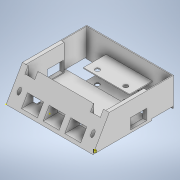
# Autodesk Inventor part: Base Onixium2
Saved by Autodesk Inventor 2021 (Build 250183000, 183)
## iProperties
Created: 2021-10-26
Part Number: Base Onixium2
Material: Genérico
Document SubType Name: Chapa
Designer: Juan Camilo
Density: 1 g/cm^3
Sheet Metal Rule: Por defecto_mm
Appearance: Valor por defecto
Author: Juan Camilo
Autodesk Inventor part; units mm, degrees
ref_plane "YZ Plane" through (0, 0, 0) normal (1, 0, 0) x (0, 1, 0)
ref_plane "XZ Plane" through (0, 0, 0) normal (0, 1, 0) x (-1, 0, 0)
ref_plane "XY Plane" through (0, 0, 0) normal (0, 0, 1) x (1, 0, 0)
sketch "Boceto2" plane through (0, 0, 0) normal (0, 1, 0) x (-1, 0, 0)
  line L0 (-49, 0) -> (49, 0)
  line L1 (49, 0) -> (49, -87)
  line L2 (49, -87) -> (-49, -87)
  line L3 (-49, -87) -> (-49, 0)
  line L4 (0, -87) -> (0, 0) construction
  circle A0 centre (-41.5, -7.5) radius 1.75
  circle A1 centre (41.5, -7.5) radius 1.75
  line L5 (-26, -87) -> (-26, -66)
  line L6 (-26, -66) -> (-49, -66)
  line L7 (26, -87) -> (26, -66)
  line L8 (26, -66) -> (49, -66)
  line L9 (49, -12) -> (-49, -12) construction
  line L10 (44.5, -24.05) -> (28.5, -24.05)
  line L11 (28.5, -24.05) -> (28.5, -13.05)
  line L12 (28.5, -13.05) -> (44.5, -13.05)
  line L13 (44.5, -13.05) -> (44.5, -24.05)
  line L14 (42.5, -23.55) -> (31.5, -23.55)
  line L15 (31.5, -14.85) -> (42.5, -14.85)
  line L16 (42.5, -14.85) -> (42.5, -23.55)
  circle A2 centre (30.2, -19.25) radius 1.05
  line L17 (31.5, -14.85) -> (31.5, -23.55)
  line L18 (-42.5, -23.55) -> (-31.5, -23.55)
  line L19 (-31.5, -14.85) -> (-42.5, -14.85)
  line L20 (-42.5, -14.85) -> (-42.5, -23.55)
  circle A3 centre (-30.2, -19.25) radius 1.05
  line L21 (-31.5, -14.85) -> (-31.5, -23.55)
  circle A4 centre (13, -21.5) radius 2.5
  circle A5 centre (-13, -21.5) radius 2.5
  circle A6 centre (16, -70) radius 2.5
  circle A7 centre (-16, -70) radius 2.5
  point P0 (26, -87)
  dimension "d6" = 3.5
  dimension "d210" = 0
  dimension "d219" = 87
  dimension "d220" = 21
  dimension "d221" = 12
  dimension "d222" = 23
  dimension "d223" = 98
  dimension "d224" = 7.5
  dimension "d225" = 7.5
  dimension "d226" = 79.5
  dimension "d229" = 2.1
  dimension "d230" = 9
  dimension "d231" = 11
  dimension "d232" = 16
  dimension "d235" = 1
  dimension "d236" = 3.6
  dimension "d239" = 2.1
  dimension "d241" = 1.3
  dimension "d242" = 5
  dimension "d243" = 36
  dimension "d244" = 9.5
  dimension "d245" = 5
  dimension "d246" = 17
  dimension "d247" = 10
  dimension "d252" = 8.7
  dimension "d254" = 4.3
  dimension "d255" = 4
  dimension "d256" = 11
  dimension "d257" = 54
  dimension "d258" = 2.85
  constraints: 44 end point, 10 symmetric about line, 8 centre point, 5 parallel, 5 point on line, 4 horizontal, 4 perpendicular, 3 midpoint, 1 equal radius, 1 vertical, 3 other
  measures "d6" diameter of A0
  measures "d210" distance of point (0, 0) L4.end
  measures "d219" distance of L1.start L1.end
  measures "d220" distance of L7.start L8.start
  measures "d221" distance between parallel lines of L0 L9
  measures "d222" distance of L8.start L8.end
  measures "d223" distance of L0.start L1.start
  measures "d224" distance from line of L1 A1.centre
  measures "d225" distance from line of L0 A1.centre
  measures "d229" diameter of L9 L12
  measures "d230" diameter of L1 L13
  measures "d231" distance of L10.end L11.end
  measures "d232" distance of L10.start L10.end
  measures "d235" diameter of L14 L10
  measures "d236" diameter of L15 L12
  measures "d239" diameter of A2
  measures "d241" distance from line of L17 A2.centre
  measures "d242" diameter of A4
  measures "d243" distance from line of L1 A4.centre
  measures "d244" distance from line of L9 A4.centre
  measures "d245" diameter of A6
  measures "d246" distance from line of L2 A6.centre
  measures "d247" distance from line of L7 A6.centre
  measures "d252" distance of L15.start L14.end
  measures "d254" distance from line of L14 A2.centre
  measures "d255" diameter of L16 L13
  measures "d256" distance of L15.start L15.end
  measures "d257" distance between parallel lines of L9 L8
  measures "d258" distance between parallel lines of L9 L15
extrude "Extrusion Base" add sketch "Boceto2" along normal blind 2 contours L0 L1 L8 L7 L2 L5 L6 L3 | L10 L11 L12 L13
sketch "Boceto4" plane through (-49, 0, -66) normal (-1, 0, 0) x (0, 0, 1)
  line L0 (66, 0) -> (0, 0) projected
  line L1 (66, 0) -> (64.8476, 2)
  line L2 (66, 0) -> (68.3082, 0) construction
  line L3 (64.8476, 2) -> (66, 2)
  line L4 (66, 0) -> (66, 2) projected
  line L5 (66, 2) -> (66, 0)
  dimension "d24" = 119.95
  constraints: 8 end point, 2 horizontal, 1 equal length, 1 perpendicular
  measures "d24" angle of L2 L1
extrude "Extrusión Angulo parte de adelante" cut sketch "Boceto4" against normal blind 100
sketch "Boceto5" plane through (0, 2, 0) normal (0, 1, 0) x (1, 0, 0)
  line L0 (49, 66) -> (26, 66) projected
  line L1 (-49, 66) -> (-49, 1.1524) projected
  line L2 (49, 66) -> (-49, 66)
  line L3 (-49, 66) -> (-49, 61.5)
  line L4 (-49, 61.5) -> (49, 61.5)
  line L5 (49, 61.5) -> (49, 66)
  point P0 (0, 0)
  dimension "d27" = 4.5
  constraints: 8 end point, 2 parallel, 1 horizontal, 1 perpendicular, 1 point on line
  measures "d27" distance of L3.end L2.end
extrude "parte trasera diseño" add sketch "Boceto5" against normal blind 0.1
sketch "Boceto10" plane through (49, 0, 0) normal (1, 0, 0) x (0, 0, -1)
  line L0 (0, 0) -> (1.1524, 2) projected
  line L1 (1.1524, 2) -> (0, 2)
  line L2 (0, 2) -> (61.5, 2)
  line L3 (61.5, 2) -> (61.5, 32)
  line L4 (61.5, 32) -> (0, 32)
  line L5 (0, 32) -> (0, 2)
  point P0 (1.1524, 2)
  constraints: 10 end point, 2 horizontal, 2 parallel, 1 perpendicular
extrude "Grado de inclinacion de 60.5 de parte delantera" add sketch "Boceto10" against normal blind 4
sketch "Boceto11" plane through (-49, 0, -66) normal (-1, 0, 0) x (0, 0, 1)
  line L0 (64.8476, 2) -> (4.5, 2) projected
  line L1 (64.8476, 2) -> (66, 2) projected
  line L2 (66, 2) -> (66, 32) projected
  line L3 (66, 32) -> (4.5, 32) projected
  line L4 (4.5, 2) -> (4.5, 32) projected
  line L5 (66, 2) -> (4.5, 2)
  line L6 (4.5, 2) -> (4.5, 32)
  line L7 (4.5, 32) -> (66, 32)
  line L8 (66, 32) -> (66, 2)
  line L9 (4.5, 32) -> (4.5, 2) projected
  point P0 (66, 0)
  point P1 (4.5, 2)
  constraints: 8 end point, 2 parallel, 1 horizontal, 1 perpendicular
extrude "Lateral derecha de diseño" add sketch "Boceto11" against normal blind 4
sketch "Boceto13" plane through (49, 0, 0) normal (1, 0, 0) x (0, 0, -1)
  line L0 (1.1524, 2) -> (0, 0) projected
  line L1 (0, 0) -> (18.438, 32)
  line L2 (0, 32) -> (61.5, 32) projected
  line L3 (0, 0) -> (36.9318, 0) construction
  line L4 (18.438, 32) -> (0, 32)
  line L5 (0, 32) -> (0, 0)
  point P0 (4, 32)
  point P1 (1.1524, 2)
  point P2 (4, 32)
  dimension "d59" = 60.05
  constraints: 8 end point, 1 collinear, 1 equal length, 1 horizontal, 1 perpendicular, 1 point on line
  measures "d59" angle of L3 L1
extrude "Lateral izquierda diseño" cut sketch "Boceto13" against normal blind 103.25
sketch "Boceto15" plane through (-45, 0, -66) normal (1, 0, 0) x (0, 0, -1)
  line L0 (-47.562, 32) -> (-66, 0) projected
  line L1 (-66, 0) -> (0, 0) projected
  line L2 (-4.5, 32) -> (-47.562, 32) projected
  line L3 (-4.5, 32) -> (-47.562, 32) projected
  line L4 (-47.562, 32) -> (-47.562, 0)
  line L5 (0, 0) -> (-66, 0) projected
  line L6 (-66, 0) -> (-47.562, 32) projected
  line L7 (-66, 0) -> (-47.562, 0)
  line L8 (-66, 0) -> (-47.562, 32)
  line L9 (0, 0) -> (0, 2) projected
  line L10 (-4.5, 2) -> (0, 2) projected
  line L11 (-4.5, 2) -> (-4.5, 32) projected
  constraints: 6 end point, 1 collinear, 1 point on line, 1 vertical
extrude "Extrusion capa parte delantera" add sketch "Boceto15" along normal blind 93 contours L4 L1 L0
sketch "Boceto17" plane through (0, 0, 0) normal (0, -1, 0) x (1, 0, 0)
  line L0 (-49, 0) -> (49, 0) projected
  line L1 (49, 0) -> (41.5, 0)
  line L2 (41.5, 0) -> (41.5, -7.5)
  line L3 (41.5, -7.5) -> (49, -7.5)
  line L4 (49, -7.5) -> (49, 0)
  circle A0 centre (41.5, -7.5) radius 1.75
  line L5 (0, 0) -> (0, -85.5)
  line L6 (-26, -85.5) -> (26, -85.5) projected
  circle A1 centre (-41.5, -7.5) radius 1.75
  dimension "d67" = 7.5
  dimension "d68" = 7.5
  dimension "d69" = 3.5
  constraints: 10 end point, 2 centre point, 2 parallel, 1 coincident, 1 horizontal, 1 midpoint, 1 perpendicular, 1 symmetric about line, 1 other
  measures "d67" distance of L3.end L2.end
  measures "d68" distance of L2.end L1.end
  measures "d69" diameter of A0
extrude "Extrusión huecos tornillos parte delantera" cut sketch "Boceto17" against normal blind 90.25 contours A0 L3 L2 | L2 L3 A0 | A1
sketch "Boceto25" plane through (-49, 0, -66) normal (-1, 0, 0) x (0, 0, 1)
  line L0 (5.5, 15) -> (23.5, 15)
  line L1 (23.5, 15) -> (23.5, 3)
  line L2 (23.5, 3) -> (5.5, 3)
  line L3 (5.5, 3) -> (5.5, 15)
  line L4 (0, 0) -> (66, 0) projected
  dimension "d131" = 3
  dimension "d132" = 18
  dimension "d133" = 12
  constraints: 8 end point, 2 parallel, 1 horizontal, 1 perpendicular
  measures "d131" distance between parallel lines of L4 L2
  measures "d132" distance of L0.start L0.end
  measures "d133" distance of L0.end L1.end
extrude "Extrusión sensores laterales" cut sketch "Boceto25" against normal blind 98.25
sketch "Boceto27" plane through (-45, 2, -18.438) normal (0, 0, -1) x (-1, 0, 0)
  line L0 (-78.5, 13) -> (-60.5, 13)
  line L1 (-60.5, 13) -> (-60.5, 1)
  line L2 (-60.5, 1) -> (-78.5, 1)
  line L3 (-78.5, 1) -> (-78.5, 13)
  line L4 (0, 0) -> (-90, 0) projected
  line L5 (-90, 0) -> (-90, 30) projected
  line L6 (-54.1, 13) -> (-36.1, 13)
  line L7 (-36.1, 13) -> (-36.1, 1)
  line L8 (-36.1, 1) -> (-54.1, 1)
  line L9 (-54.1, 1) -> (-54.1, 13)
  line L10 (-29.7, 13) -> (-11.7, 13)
  line L11 (-11.7, 13) -> (-11.7, 1)
  line L12 (-11.7, 1) -> (-29.7, 1)
  line L13 (-29.7, 1) -> (-29.7, 13)
  point P0 (-45, -2)
  point P1 (-13.5, 0)
  point P2 (-76.5, 0)
  dimension "d144" = 18
  dimension "d145" = 12
  dimension "d146" = 1
  dimension "d147" = 11.5
  dimension "d148" = 1
  dimension "d149" = 12
  dimension "d150" = 18
  dimension "d151" = 6.4
  dimension "d152" = 6.4
  dimension "d153" = 1
  dimension "d154" = 18
  dimension "d155" = 12
  constraints: 24 end point, 6 parallel, 3 horizontal, 3 perpendicular
  measures "d144" distance of L0.start L0.end
  measures "d145" distance of L0.end L1.end
  measures "d146" distance between parallel lines of L4 L2
  measures "d147" distance between parallel lines of L5 L3
  measures "d148" distance between parallel lines of L4 L8
  measures "d149" distance of L8.end L6.start
  measures "d150" distance of L6.start L6.end
  measures "d151" distance between parallel lines of L9 L1
  measures "d152" distance between parallel lines of L7 L13
  measures "d153" distance between parallel lines of L4 L12
  measures "d154" distance of L10.start L10.end
  measures "d155" distance of L10.end L11.end
extrude "Extrusión sensores delanteros" cut sketch "Boceto27" against normal blind 19.25
sketch "Boceto39" plane through (0, 2, 0) normal (0, 1, 0) x (1, 0, 0)
  line L0 (-42.5, 23.55) -> (-31.5, 23.55)
  line L1 (-31.5, 23.55) -> (-31.5, 14.8119)
  line L2 (-31.5, 14.8119) -> (-42.5, 14.8119)
  line L3 (-42.5, 14.8119) -> (-42.5, 23.55)
  circle A0 centre (-30.2, 19.25) radius 1.1
  line L4 (0, 64) -> (0, 18.438)
  line L5 (-29.5343, 18.438) -> (29.5343, 18.438) projected
  line L6 (42.5, 23.55) -> (31.5, 23.55)
  line L7 (31.5, 23.55) -> (31.5, 14.8119)
  line L8 (31.5, 14.8119) -> (42.5, 14.8119)
  line L9 (42.5, 14.8119) -> (42.5, 23.55)
  circle A1 centre (30.2, 19.25) radius 1.1
  arc A2 (-29.5343, 18.438) -> (-30.8657, 18.438) centre (-30.2, 19.25) ccw projected
  point P0 (0, 0)
  dimension "d259" = 11
  dimension "d262" = 2.2
  dimension "d263" = 1.3
  dimension "d264" = 4.3
  dimension "d270" = 2.15
  constraints: 18 end point, 5 symmetric about line, 2 centre point, 2 parallel, 1 horizontal, 1 midpoint, 1 perpendicular, 1 other
  measures "d259" distance of L0.start L0.end
  measures "d262" diameter of A0
  measures "d263" distance from line of L1 A0.centre
  measures "d264" distance from line of L0 A0.centre
extrude "Extrusión arreglo sensores" cut sketch "Boceto39" along normal mid plane 85.25
sketch "Boceto40" plane through (0, 2, 0) normal (0, 1, 0) x (1, 0, 0)
  line L0 (-30.65, 14.8119) -> (-31.5, 14.8119)
  line L1 (0, 64) -> (0, 18.438)
  line L2 (-29.5343, 18.438) -> (29.5343, 18.438) projected
  line L3 (31.5, 23.55) -> (31.5, 14.8119)
  line L4 (31.5, 23.55) -> (30.65, 23.55)
  line L5 (30.65, 23.55) -> (30.65, 14.8119)
  line L6 (30.65, 14.8119) -> (31.5, 14.8119)
  line L7 (-31.5, 23.55) -> (-28.1, 23.55)
  line L8 (-28.1, 23.55) -> (-28.1, 14.8119)
  line L9 (-28.1, 14.8119) -> (-31.5, 14.8119)
  line L10 (-31.5, 14.8119) -> (-31.5, 23.55)
  arc A0 (-29.4579, 18.438) -> (-30.9421, 18.438) centre (-30.2, 19.25) ccw projected
  line L11 (31.5, 23.55) -> (28.1, 23.55)
  line L12 (28.1, 23.55) -> (28.1, 14.8119)
  line L13 (28.1, 14.8119) -> (31.5, 14.8119)
  line L14 (31.5, 14.8119) -> (31.5, 23.55)
  point P0 (0, 0)
  point P1 (-31.5, 14.8119)
  point P2 (31.5, 14.8119)
  dimension "d271" = 1
  constraints: 28 end point, 7 symmetric about line, 2 parallel, 1 horizontal, 1 midpoint, 1 perpendicular
  measures "d271" distance edge to line of A0 L8
extrude "Extrusión desnivel sensores" cut sketch "Boceto40" along normal mid plane 2
sketch "Boceto placa" plane through (0, 2, 0) normal (0, 1, 0) x (1, 0, 0)
  circle A0 centre (-32, 31.5) radius 1.75 projected
  circle A1 centre (31.5, 58) radius 1.75 projected
  line L0 (-32, 31.5) -> (31.5, 31.5)
  line L1 (31.5, 31.5) -> (31.5, 58)
  line L2 (31.5, 58) -> (-32, 58)
  line L3 (-32, 58) -> (-32, 31.5)
  line L4 (-42, 27.507) -> (42, 27.507)
  line L5 (42, 27.507) -> (42, 63.007)
  line L6 (42, 63.007) -> (-42, 63.007)
  line L7 (-42, 63.007) -> (-42, 27.507)
  line L8 (-45, 61.5) -> (-45, 18.438) projected
  line L9 (45, 18.438) -> (45, 61.5) projected
  line L10 (-22.385, 61.5) -> (-45, 61.5) projected
  line L11 (-45, 18.438) -> (45, 18.438) projected
  point P0 (0, 0)
  dimension "d167" = 63.5
  dimension "d168" = 26.5
  dimension "d172" = 84
  dimension "d176" = 10
  dimension "d177" = 3.993
  dimension "d178" = 3.5
  dimension "d179" = 35.5
  dimension "d180" = 9.069
  constraints: 16 end point, 4 parallel, 2 horizontal, 2 perpendicular
  measures "d167" distance of L0.start L0.end
  measures "d168" distance of L2.end L0.start
  measures "d172" distance of L4.start L4.end
  measures "d176" distance from line of L7 L0.start
  measures "d177" distance from line of L4 L0.start
  measures "d178" diameter of A0
  measures "d179" distance between parallel lines of L6 L4
  measures "d180" distance between parallel lines of L11 L4
sketch "Boceto48" plane through (0, 2, 0) normal (0, 1, 0) x (1, 0, 0)
  line L0 (26, 87) -> (-26, 87) projected
  line L1 (-26, 66) -> (26, 66)
  line L2 (26, 66) -> (26, 87)
  line L3 (26, 87) -> (-26, 87)
  line L4 (-26, 87) -> (-26, 66)
  point P0 (0, 0)
  point P1 (-26, 87)
  constraints: 8 end point, 2 parallel, 1 horizontal, 1 perpendicular
extrude "Extrusión35" cut sketch "Boceto48" against normal blind 1
sketch "Boceto49" plane through (49, 0, -66) normal (1, 0, 0) x (0, 0, -1)
  line L0 (-4.5, 2) -> (-4.5, 32) projected
  line L1 (-4.5, 2) -> (24, 2)
  line L2 (24, 2) -> (24, 32)
  line L3 (24, 32) -> (-4.5, 32)
  line L4 (-4.5, 32) -> (-4.5, 2)
  point P0 (-66, 0)
  dimension "d281" = 28.5
  constraints: 8 end point, 2 parallel, 1 horizontal, 1 perpendicular
  measures "d281" distance between parallel lines of L2 L0
extrude "Extrusión36" add sketch "Boceto49" against normal blind 1
sketch "Boceto50" plane through (-49, 0, -66) normal (-1, 0, 0) x (0, 0, 1)
  line L0 (4.5, 32) -> (4.5, 2) projected
  line L1 (4.5, 32) -> (-24, 32)
  line L2 (-24, 32) -> (-24, 2)
  line L3 (-24, 2) -> (4.5, 2)
  line L4 (4.5, 2) -> (4.5, 32)
  point P0 (66, 0)
  dimension "d284" = 28.5
  constraints: 8 end point, 2 parallel, 1 horizontal, 1 perpendicular
  measures "d284" distance between parallel lines of L0 L2
extrude "Extrusión37" add sketch "Boceto50" against normal blind 1
sketch "Boceto52" plane through (26, 0, -87) normal (0, 0, -1) x (-1, 0, 0)
  line L0 (0, 1) -> (52, 1) projected
  line L1 (0, 0) -> (52, 0)
  line L2 (52, 0) -> (52, 1)
  line L3 (52, 1) -> (0, 1)
  line L4 (0, 1) -> (0, 0)
  point P0 (26, 0)
  constraints: 8 end point, 2 parallel, 1 horizontal, 1 perpendicular
sketch "Boceto53" plane through (26, 0, -87) normal (0, 0, -1) x (-1, 0, 0)
  line L0 (52, 1) -> (0, 1) projected
  line L1 (52, 0) -> (75, 0) projected
  line L2 (0, 1) -> (52, 1)
  line L3 (52, 1) -> (52, 0)
  line L4 (52, 0) -> (0, 0)
  line L5 (0, 0) -> (0, 1)
  point P0 (26, 0)
  constraints: 8 end point, 2 parallel, 1 horizontal, 1 perpendicular
extrude "Extrusión39" add sketch "Boceto53" along normal blind 3
sketch "Boceto54" plane through (26, 0, -90) normal (0, 0, -1) x (-1, 0, 0)
  point P0 (26, 0)
sketch "Boceto55" plane through (26, 0, -90) normal (0, 0, -1) x (-1, 0, 0)
  line L0 (-23, 0) -> (0, 0) projected
  line L1 (75, 32) -> (75, 2) projected
  line L2 (-23, 0) -> (75, 0)
  line L3 (75, 0) -> (75, 32)
  line L4 (75, 32) -> (-23, 32)
  line L5 (-23, 32) -> (-23, 0)
  point P0 (26, 0)
  constraints: 8 end point, 2 parallel, 1 horizontal, 1 perpendicular
extrude "Extrusión40" add sketch "Boceto55" along normal blind 1
sketch "Boceto56" plane through (26, 0, -90) normal (0, 0, 1) x (1, 0, 0)
  line L0 (-52, 15.5) -> (0, 15.5)
  line L1 (0, 15.5) -> (0, 14.5)
  line L2 (0, 14.5) -> (-52, 14.5)
  line L3 (-52, 14.5) -> (-52, 15.5)
  line L4 (-52, 1) -> (0, 1) projected
  point P0 (-26, 0)
  dimension "d293" = 13.5
  dimension "d294" = 1
  dimension "d295" = 0
  dimension "d296" = 0
  constraints: 8 end point, 2 parallel, 1 horizontal, 1 perpendicular
  measures "d293" distance between parallel lines of L4 L2
  measures "d294" distance between parallel lines of L0 L2
  measures "d295" distance from line of L4.start L3
  measures "d296" distance from line of L4.end L1
extrude "Extrusión41" add sketch "Boceto56" along normal blind 25.75
sketch "Boceto57" plane through (-26, 14.5, -90) normal (0, -1, 0) x (1, 0, 0)
  circle A0 centre (10, 20) radius 2.5 projected
  circle A1 centre (10, 20) radius 2.5
  circle A2 centre (42, 20) radius 2.5 projected
  circle A3 centre (42, 20) radius 2.5
  point P0 (26, 90)
  constraints: 2 centre point, 2 coincident
extrude "Extrusión42" cut sketch "Boceto57" against normal blind 25.75
sketch "Boceto58" plane through (-26, 15.5, -90) normal (0, 1, 0) x (1, 0, 0)
  point P0 (26, -90)
sketch "Boceto59" plane through (-49, 0, -66) normal (-1, 0, 0) x (0, 0, 1)
  point P0 (66, 0)
equation "\"Radio_pliegue\" = Grosor"
equation "\"Anchura_desahogo_plegado\" = Grosor"
equation "\"Profundidad_desahogo_plegado\" = 0.5 * Grosor"
equation "\"Tamaño_destalonado\" = 4 * Grosor"
equation "\"Remanente_mínimo\" = 2 * Grosor"
equation "\"Radiodetransición\" = Radio_pliegue"
equation "\"Tamaño_de_radio_de_Jacobi\" = Radio_pliegue"
equation "\"TamañoSeparación\" = Grosor"
equation "\"Grosor\" = 0.5"
